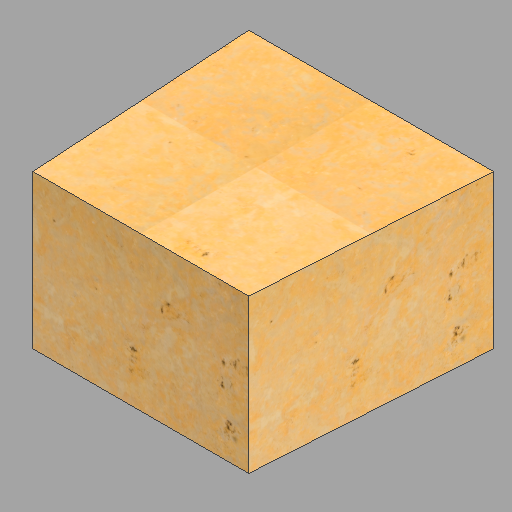
# Autodesk Inventor part: E1
Saved by Autodesk Inventor 2023 (Build 270158030, 158C)
## iProperties
RuleStatus: InUse
Created: 2022-05-23
Part Number: E1
Material: Granite, Cut, Polished
Document SubType Name: Modeling
Designer: awelt
Mass: 1.37599e+06 g
Surface Area: 39036.9 cm^2
Volume: 509626 cm^3
Density: 2.7 g/cm^3
Appearance: Amber Select
AfterDocSave0: Convert in3 volume to ft3
in3 to ft3: 0.01
TEST: 0.01
Author: awelt
Autodesk Inventor part; units mm, degrees
ref_plane "YZ Plane" through (0, 0, 0) normal (1, 0, 0) x (0, 1, 0)
ref_plane "XZ Plane" through (0, 0, 0) normal (0, 1, 0) x (-1, 0, 0)
ref_plane "XY Plane" through (0, 0, 0) normal (0, 0, 1) x (1, 0, 0)
sketch "Sketch1" plane through (0, 0, 0) normal (0, 1, 0) x (-1, 0, 0)
  line L0 (0, 0) -> (-971.55, 0)
  line L1 (-57.2888, 914.4) -> (-914.2612, 914.4)
  line L2 (0, 0) -> (-57.2888, 914.4)
  line L3 (-971.55, 0) -> (-914.2612, 914.4)
  line L4 (-485.775, 0) -> (-485.775, 914.4) construction
  dimension "d0" = 971.55
  dimension "d2" = 914.4
  dimension "d3" = 7.17
  dimension "d4" = 57.2888
  dimension "d5" = 57.2888
  constraints: 10 end point, 2 horizontal, 2 midpoint, 1 other
  measures "d0" distance of L0.start L0.end
  measures "d2" distance between parallel lines of L1 L0
  measures "d3" angle of L3 L2
  measures "d4" horizontal distance of L1.start L0.start
  measures "d5" horizontal distance of L1.end L0.end
extrude "Extrusion1" add sketch "Sketch1" along normal blind 609.6
